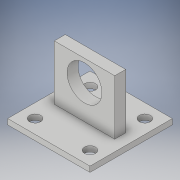
# Autodesk Inventor part: pneumatics front holder
Saved by Autodesk Inventor 2018 (Build 220112000, 112)
## iProperties
Created: 2019-01-16
Part Number: pneumatics front holder
Material: Generic
Document SubType Name: Modeling
Designer: s-4008082
Density: 1 g/cm^3
Appearance: Default
Author: s-4008082
Autodesk Inventor part; units mm, degrees
ref_plane "YZ Plane" through (0, 0, 0) normal (1, 0, 0) x (0, 1, 0)
ref_plane "XZ Plane" through (0, 0, 0) normal (0, 1, 0) x (-1, 0, 0)
ref_plane "XY Plane" through (0, 0, 0) normal (0, 0, 1) x (1, 0, 0)
sketch "Sketch1" plane through (0, 0, 0) normal (0, 1, 0) x (-1, 0, 0)
  line L0 (-19.05, -19.05) -> (19.05, -19.05)
  line L1 (19.05, -19.05) -> (19.05, 19.05)
  line L2 (19.05, 19.05) -> (-19.05, 19.05)
  line L3 (-19.05, 19.05) -> (-19.05, -19.05)
  line L4 (-19.05, -19.05) -> (19.05, 19.05) construction
  line L5 (19.05, -19.05) -> (-19.05, 19.05) construction
  point P0 (0, 0)
  dimension "d0" = 38.1
  dimension "d1" = 38.1
  constraints: 12 end point, 2 midpoint, 2 parallel, 1 horizontal, 1 perpendicular
  measures "d0" distance of L0.end L1.end
  measures "d1" distance of L1.end L2.end
extrude "Extrusion1" add sketch "Sketch1" along normal blind 2.54
sketch "Sketch2" plane through (0, 2.54, 0) normal (0, 1, 0) x (1, 0, 0)
  line L0 (13.97, -2.54) -> (-13.97, -2.54)
  line L1 (-13.97, -2.54) -> (-13.97, 2.54)
  line L2 (-13.97, 2.54) -> (13.97, 2.54)
  line L3 (13.97, 2.54) -> (13.97, -2.54)
  line L4 (-19.05, 19.05) -> (-19.05, -19.05) projected
  line L5 (19.05, -19.05) -> (19.05, 19.05) projected
  line L6 (19.05, 19.05) -> (-19.05, 19.05) projected
  point P0 (0, 0)
  dimension "d4" = 5.08
  dimension "d5" = 5.08
  dimension "d6" = 16.51
  dimension "d7" = 5.08
  constraints: 8 end point, 2 parallel, 1 horizontal, 1 perpendicular
  measures "d4" distance between parallel lines of L4 L1
  measures "d5" distance between parallel lines of L5 L3
  measures "d6" distance between parallel lines of L6 L2
  measures "d7" distance between parallel lines of L2 L0
extrude "Extrusion2" add sketch "Sketch2" along normal blind 25.4
sketch "Sketch3" plane through (-13.97, 2.54, 2.54) normal (0, 0, 1) x (1, 0, 0)
  circle A0 centre (13.97, 15.5704) radius 8.0645
  point P0 (13.97, -2.54)
  dimension "d10" = 16.129
  constraints: 1 centre point
  measures "d10" diameter of A0
extrude "Extrusion3" cut sketch "Sketch3" against normal blind 50.8
sketch "Sketch4" plane through (0, 2.54, 0) normal (0, 1, 0) x (1, 0, 0)
  circle A0 centre (-12.7, -12.7) radius 2.5797
  circle A1 centre (-12.7, 12.7) radius 2.5797
  circle A2 centre (12.7, 12.7) radius 2.5797
  circle A3 centre (12.7, -12.7) radius 2.5797
  line L0 (-19.05, 19.05) -> (-19.05, -19.05) projected
  line L1 (-19.05, -19.05) -> (19.05, -19.05) projected
  line L2 (19.05, -19.05) -> (19.05, 19.05) projected
  line L3 (19.05, 19.05) -> (-19.05, 19.05) projected
  point P0 (0, 0)
  dimension "d13" = 5.1594
  dimension "d14" = 5.1594
  dimension "d15" = 5.1594
  dimension "d16" = 5.1594
  dimension "d17" = 6.35
  dimension "d18" = 6.35
  dimension "d19" = 6.35
  dimension "d20" = 6.35
  dimension "d21" = 6.35
  dimension "d22" = 6.35
  dimension "d23" = 6.35
  dimension "d24" = 6.35
  constraints: 4 centre point
  measures "d13" diameter of A0
  measures "d14" diameter of A3
  measures "d15" diameter of A2
  measures "d16" diameter of A1
  measures "d17" distance from line of L0 A0.centre
  measures "d18" distance from line of L1 A0.centre
  measures "d19" distance from line of L1 A3.centre
  measures "d20" distance from line of L2 A3.centre
  measures "d21" distance from line of L0 A1.centre
  measures "d22" distance from line of L3 A1.centre
  measures "d23" distance from line of L2 A2.centre
  measures "d24" distance from line of L3 A2.centre
extrude "Extrusion4" cut sketch "Sketch4" against normal blind 50.8 contours A0 | A1 | A2 | A3
equation "\"d1\" = d0"
equation "\"d4\" = d5"
equation "\"d14\" = d13"
equation "\"d15\" = d13"
equation "\"d16\" = d13"
equation "\"d18\" = d17"
equation "\"d19\" = d17"
equation "\"d20\" = d17"
equation "\"d21\" = d17"
equation "\"d22\" = d17"
equation "\"d23\" = d17"
equation "\"d24\" = d17"
body "Solid1"
